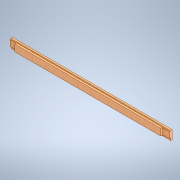
# Autodesk Inventor part: bottomv2
Saved by Autodesk Inventor 2020 (Build 240168000, 168)
## iProperties
Created: 2020-05-19
Part Number: bottomv2
Material: Wood (Cherry)
Document SubType Name: Modeling
Designer: kolbe
Density: 0.63 g/cm^3
Appearance: Cherry - Natural Low Gloss
Author: kolbe
Autodesk Inventor part; units mm, degrees
ref_plane "YZ Plane" through (0, 0, 0) normal (1, 0, 0) x (0, 1, 0)
ref_plane "XZ Plane" through (0, 0, 0) normal (0, 1, 0) x (-1, 0, 0)
ref_plane "XY Plane" through (0, 0, 0) normal (0, 0, 1) x (1, 0, 0)
sketch "Sketch1" plane through (0, 0, 0) normal (0, 0, 1) x (1, 0, 0)
  line L0 (0, 0) -> (889, 0)
  line L1 (889, 0) -> (889, 50.8)
  line L2 (889, 50.8) -> (0, 50.8)
  line L3 (0, 50.8) -> (0, 0)
  dimension "d0" = 889
  dimension "d1" = 50.8
  constraints: 8 end point, 2 parallel, 1 horizontal, 1 perpendicular
  measures "d0" distance of L2.end L1.end
  measures "d1" distance of L1.end L0.end
extrude "Extrusion1" add sketch "Sketch1" along normal blind 25.4
sketch "Sketch2" plane through (0, 0, 25.4) normal (0, 0, 1) x (1, 0, 0)
  line L0 (0, 0) -> (889, 0)
  line L1 (889, 0) -> (889, 12.7)
  line L2 (889, 12.7) -> (0, 12.7)
  line L3 (0, 12.7) -> (0, 0)
  dimension "d4" = 889
  dimension "d5" = 12.7
  constraints: 8 end point, 2 parallel, 1 horizontal, 1 perpendicular
  measures "d4" distance of L2.end L1.end
  measures "d5" distance of L1.end L0.end
extrude "Extrusion2" cut sketch "Sketch2" against normal blind 19.05
sketch "Sketch3" plane through (0, 0, 25.4) normal (0, 0, 1) x (1, 0, 0)
  line L0 (0, 50.8) -> (0, 0) projected
  line L1 (0, 50.8) -> (38.1, 50.8)
  line L2 (38.1, 50.8) -> (38.1, 12.7)
  line L3 (38.1, 12.7) -> (0, 12.7)
  line L4 (0, 12.7) -> (0, 50.8)
  dimension "d8" = 38.1
  dimension "d9" = 38.1
  constraints: 8 end point, 2 parallel, 1 horizontal, 1 perpendicular
  measures "d8" distance of L2.end L3.end
  measures "d9" distance of L1.end L2.end
extrude "Extrusion3" cut sketch "Sketch3" against normal blind 12.7
sketch "Sketch4" plane through (0, 0, 25.4) normal (0, 0, 1) x (1, 0, 0)
  line L0 (889, 50.8) -> (850.9, 50.8)
  line L1 (850.9, 50.8) -> (850.9, 12.7)
  line L2 (850.9, 12.7) -> (889, 12.7)
  line L3 (889, 12.7) -> (889, 50.8)
  point P0 (0, 0)
  dimension "d12" = 38.1
  dimension "d13" = 38.1
  constraints: 8 end point, 2 parallel, 1 horizontal, 1 perpendicular
  measures "d12" distance of L2.end L1.end
  measures "d13" distance of L1.end L0.end
extrude "Extrusion4" cut sketch "Sketch4" against normal blind 12.7
sketch "Sketch5" plane through (0, 50.8, 0) normal (0, 1, 0) x (1, 0, 0)
  line L0 (0, -6.35) -> (0, -12.7) projected
  line L1 (0, -12.7) -> (0, -15.875)
  line L2 (0, -15.875) -> (889, -15.875)
  line L3 (889, -15.875) -> (889, -9.525)
  line L4 (889, -12.7) -> (889, -6.35) projected
  line L5 (889, -9.525) -> (0, -9.525)
  line L6 (0, -9.525) -> (0, -12.7)
  dimension "d22" = 3.175
  dimension "d23" = 889
  dimension "d24" = 889
  constraints: 10 end point, 1 midpoint, 1 perpendicular, 1 point on line, 1 vertical
  measures "d22" distance of L0.end L1.end
  measures "d23" distance of L1.end L2.end
  measures "d24" distance of L3.end L5.end
extrude "Extrusion5" cut sketch "Sketch5" against normal blind 6.35
body "Solid1"
